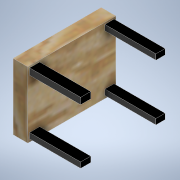
# Autodesk Inventor part: TABLE NEW
Saved by Autodesk Inventor 2021 (Build 250183000, 183)
## iProperties
Created: 2021-07-11
Part Number: TABLE NEW
Material: Generic
Document SubType Name: Modeling
Designer: HP
Density: 1 g/cm^3
Appearance: Glossy - Black
Author: HP
Autodesk Inventor part; units mm, degrees
ref_plane "YZ Plane" through (0, 0, 0) normal (1, 0, 0) x (0, 1, 0)
ref_plane "XZ Plane" through (0, 0, 0) normal (0, 1, 0) x (-1, 0, 0)
ref_plane "XY Plane" through (0, 0, 0) normal (0, 0, 1) x (1, 0, 0)
sketch "Sketch1" plane through (0, 0, 0) normal (1, 0, 0) x (0, 1, 0)
  line L0 (22.225, 104.775) -> (136.525, 104.775)
  line L1 (136.525, 104.775) -> (136.525, -47.625)
  line L2 (136.525, -47.625) -> (22.225, -47.625)
  line L3 (22.225, -47.625) -> (22.225, 104.775)
  point P0 (0, 0)
  dimension "d0" = 114.3
  dimension "d1" = 152.4
  constraints: 8 end point, 2 parallel, 1 horizontal, 1 perpendicular
  measures "d0" distance of L1.end L2.end
  measures "d1" distance of L0.end L1.end
extrude "Extrusion1" add sketch "Sketch1" along normal blind 7.62
sketch "Sketch2" plane through (7.62, 0, 0) normal (1, 0, 0) x (0, 0, -1)
  line L0 (-101.6, 133.35) -> (-84.1375, 133.35)
  line L1 (-84.1375, 133.35) -> (-84.1375, 122.2375)
  line L2 (-84.1375, 122.2375) -> (-101.6, 122.2375)
  line L3 (-101.6, 122.2375) -> (-101.6, 133.35)
  line L4 (-101.6, 26.9875) -> (-84.1375, 26.9875)
  line L5 (-84.1375, 26.9875) -> (-84.1375, 36.5125)
  line L6 (-84.1375, 36.5125) -> (-101.6, 36.5125)
  line L7 (-101.6, 36.5125) -> (-101.6, 26.9875)
  line L8 (44.45, 133.35) -> (28.575, 133.35)
  line L9 (28.575, 133.35) -> (28.575, 123.825)
  line L10 (28.575, 123.825) -> (44.45, 123.825)
  line L11 (44.45, 123.825) -> (44.45, 133.35)
  line L12 (44.45, 26.9875) -> (28.575, 26.9875)
  line L13 (28.575, 26.9875) -> (28.575, 36.5125)
  line L14 (28.575, 36.5125) -> (44.45, 36.5125)
  line L15 (44.45, 36.5125) -> (44.45, 26.9875)
  point P0 (0, 0)
  constraints: 32 end point, 8 parallel, 5 point on line, 4 horizontal, 4 perpendicular
extrude "Extrusion2" add sketch "Sketch2" along normal blind 88.265
sketch "Sketch3" plane through (0, 0, 0) normal (-1, 0, 0) x (0, 0, 1)
  line L0 (-47.625, 22.225) -> (-47.625, 136.525) projected
  line L1 (-47.625, 136.525) -> (104.775, 136.525) projected
  line L2 (-47.625, 22.225) -> (-39.6875, 22.225)
  line L3 (-39.6875, 22.225) -> (-39.6875, 136.525)
  line L4 (-39.6875, 136.525) -> (-47.625, 136.525)
  line L5 (-47.625, 136.525) -> (-47.625, 22.225)
  line L6 (104.775, 136.525) -> (104.775, 22.225) projected
  line L7 (-47.625, 136.525) -> (104.775, 136.525)
  line L8 (104.775, 136.525) -> (104.775, 128.5875)
  line L9 (-47.625, 128.5875) -> (-47.625, 136.525)
  line L10 (104.775, 22.225) -> (-47.625, 22.225) projected
  line L11 (104.775, 136.525) -> (96.8375, 136.525)
  line L12 (96.8375, 22.225) -> (104.775, 22.225)
  line L13 (104.775, 22.225) -> (104.775, 136.525)
  line L14 (-47.625, 22.225) -> (104.775, 22.225)
  line L15 (104.775, 22.225) -> (104.775, 30.1625)
  line L16 (104.775, 30.1625) -> (-47.625, 30.1625)
  line L17 (-47.625, 30.1625) -> (-47.625, 22.225)
  line L18 (-47.625, 136.525) -> (104.775, 136.525)
  line L19 (104.775, 136.525) -> (104.775, 128.5875)
  line L20 (104.775, 128.5875) -> (-47.625, 128.5875)
  line L21 (-47.625, 128.5875) -> (-47.625, 136.525)
  point P0 (0, 0)
  constraints: 36 end point, 8 parallel, 5 horizontal, 4 perpendicular, 4 point on line
extrude "Extrusion3" add sketch "Sketch3" along normal blind 17.78
sketch "Sketch4" plane through (7.62, 22.225, -47.625) normal (0, -1, 0) x (1, 0, 0)
  point P0 (-7.62, 47.625)
body "Solid1"
